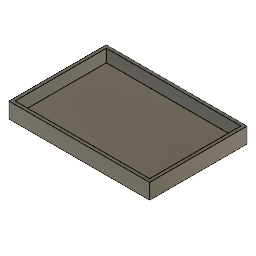
BlimpBagBreadMount v3 (Autodesk Fusion 360 design; units mm, degrees)
Autodesk Fusion 360 part; units mm, degrees
sketch "Sketch1" plane through (0, 0, 0) normal (0, 0, 1) x (1, 0, 0)
  line L0 (0, 0) -> (85.5, 0)
  line L1 (85.5, 0) -> (85.5, 58)
  line L2 (85.5, 58) -> (0, 58)
  line L3 (0, 58) -> (0, 0)
  line L4 (87.5, -2) -> (87.5, 60)
  line L5 (87.5, 60) -> (-2, 60)
  line L6 (-2, 60) -> (-2, -2)
  line L7 (-2, -2) -> (87.5, -2)
  dimension "d1" = 85.5
  dimension "d2" = 58
  dimension "d3" = 2
  constraint horizontal L0
  constraint vertical L1
  constraint horizontal L2
  constraint vertical L3
  constraint coincident L0.start L3.end
  measures "d1" distance of L0.start L0.end
  measures "d2" distance of L0.start L2.end
extrude "Extrude1" add sketch "Sketch1" along normal blind 10
sketch "Sketch2" plane through (0, 0, 0) normal (0, 0, 1) x (1, 0, 0)
  line L0 (0, 0) -> (85.5, 0)
  line L1 (85.5, 0) -> (85.5, 58)
  line L2 (85.5, 58) -> (0, 58)
  line L3 (0, 58) -> (0, 0)
  point P0 (85.5, 58)
  constraint horizontal L0
  constraint vertical L1
  constraint horizontal L2
  constraint vertical L3
  constraint coincident P0 L1.end
  constraint coincident L0.start L3.end
extrude "Extrude2" add sketch "Sketch2" along normal blind 2
sketch "Sketch3" plane through (0, 0, 0) normal (0, 0, -1) x (1, 0, 0)
  line L0 (87.5, 2) -> (-2, 2)
  line L1 (-2, 2) -> (-2, -60)
  line L2 (-2, -60) -> (87.5, -60)
  line L3 (87.5, -60) -> (87.5, 2)
  line L4 (-2, -29) -> (87.5, -29)
  circle A0 centre (13, -9) radius 1.125
  circle A1 centre (13, -49) radius 1.125
  dimension "d8" = 2.25
  dimension "d9" = 2.25
  dimension "d10" = 20
  dimension "d11" = 20
  dimension "d14" = 15
  constraint midpoint L1 L4.start
  constraint midpoint L3 L4.end
  measures "d8" diameter of A0
  measures "d9" diameter of A1
  measures "d10" distance of L4 A0.centre
  measures "d11" distance of L4 A1.centre
  measures "d14" distance of L1 A1.centre
extrude "Extrude3" add sketch "Sketch3" along normal blind 6 contours A0 | A1
sketch "Sketch4" plane through (0, 0, 0) normal (0, 0, -1) x (1, 0, 0)
  circle A0 centre (13, -9) radius 1.125
  circle A1 centre (13, -49) radius 1.125
  line L0 (87.5, 2) -> (-2, 2)
  line L1 (-2, 2) -> (-2, -60)
  line L2 (-2, -60) -> (87.5, -60)
  line L3 (87.5, -60) -> (87.5, 2)
